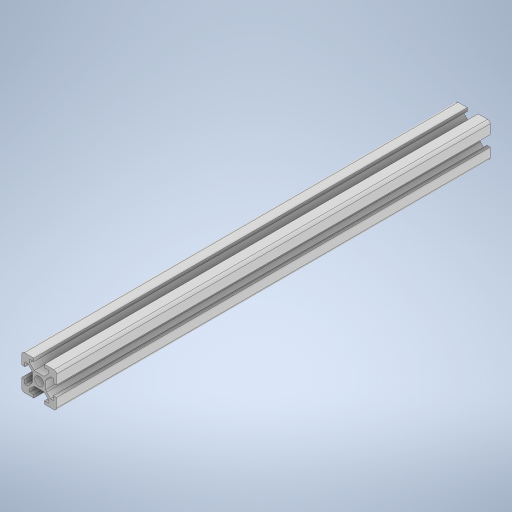
# Autodesk Inventor part: perfil_2020T
Saved by Autodesk Inventor 2023.2 (Build 272271030, 271C)
## iProperties
Created: 2023-03-04
Part Number: perfil_2020T
Material: Generic
Document SubType Name: Modeling
Designer: Cris Pat
Density: 1 g/cm^3
Appearance: Default
Author: Cris Pat
Autodesk Inventor part; units mm, degrees
ref_plane "YZ Plane" through (0, 0, 0) normal (1, 0, 0) x (0, 1, 0)
ref_plane "XZ Plane" through (0, 0, 0) normal (0, 1, 0) x (-1, 0, 0)
ref_plane "XY Plane" through (0, 0, 0) normal (0, 0, 1) x (1, 0, 0)
sketch "Sketch1" plane through (0, 0, 0) normal (0, 0, 1) x (1, 0, 0)
  line L0 (-10, 10) -> (10, 10) construction
  line L1 (10, 10) -> (10, -10) construction
  line L2 (10, -10) -> (-10, -10) construction
  line L3 (-10, -10) -> (-10, 10) construction
  line L4 (0, 10) -> (0, -10) construction
  circle A0 centre (0, 0) radius 2.5
  line L5 (10, 0) -> (-10, 0) construction
  line L6 (0, 0) -> (10, 10) construction
  line L7 (-3.9, 3.9) -> (3.9, 3.9) construction
  line L8 (3.9, 3.9) -> (3.9, -3.9) construction
  line L9 (3.9, -3.9) -> (-3.9, -3.9) construction
  line L10 (-3.9, -3.9) -> (-3.9, 3.9) construction
  line L11 (2.8393, 3.9) -> (3.9, 2.8393) construction
  line L12 (10, 10) -> (5.5, 10) construction
  line L13 (5.5, 10) -> (5.5, 5.5) construction
  line L14 (5.5, 5.5) -> (10, 5.5) construction
  line L15 (10, 5.5) -> (10, 10) construction
  line L16 (3.9, 0) -> (3.9, 2.8393)
  line L17 (3.9, 2.8393) -> (6.5607, 5.5)
  line L18 (0, 3.9) -> (2.8393, 3.9)
  line L19 (2.8393, 3.9) -> (5.5, 6.5607)
  line L20 (10, 10) -> (10, 3.1)
  line L21 (10, 3.1) -> (8.2, 3.1)
  line L22 (8.2, 3.1) -> (8.2, 5.5)
  line L23 (6.5607, 5.5) -> (8.2, 5.5)
  line L24 (10, 10) -> (3.1, 10)
  line L25 (3.1, 10) -> (3.1, 8.2)
  line L26 (3.1, 8.2) -> (5.5, 8.2)
  line L27 (5.5, 6.5607) -> (5.5, 8.2)
  line L28 (-3.9, 0) -> (-3.9, 2.8393)
  line L29 (-3.9, 2.8393) -> (-6.5607, 5.5)
  line L30 (0, 3.9) -> (-2.8393, 3.9)
  line L31 (-2.8393, 3.9) -> (-5.5, 6.5607)
  line L32 (-10, 10) -> (-10, 3.1)
  line L33 (-10, 3.1) -> (-8.2, 3.1)
  line L34 (-8.2, 3.1) -> (-8.2, 5.5)
  line L35 (-6.5607, 5.5) -> (-8.2, 5.5)
  line L36 (-10, 10) -> (-3.1, 10)
  line L37 (-3.1, 10) -> (-3.1, 8.2)
  line L38 (-3.1, 8.2) -> (-5.5, 8.2)
  line L39 (-5.5, 6.5607) -> (-5.5, 8.2)
  line L40 (3.9, 0) -> (3.9, -2.8393)
  line L41 (3.9, -2.8393) -> (6.5607, -5.5)
  line L42 (0, -3.9) -> (2.8393, -3.9)
  line L43 (2.8393, -3.9) -> (5.5, -6.5607)
  line L44 (10, -10) -> (10, -3.1)
  line L45 (10, -3.1) -> (8.2, -3.1)
  line L46 (8.2, -3.1) -> (8.2, -5.5)
  line L47 (6.5607, -5.5) -> (8.2, -5.5)
  line L48 (10, -10) -> (3.1, -10)
  line L49 (3.1, -10) -> (3.1, -8.2)
  line L50 (3.1, -8.2) -> (5.5, -8.2)
  line L51 (5.5, -6.5607) -> (5.5, -8.2)
  line L52 (-3.9, 0) -> (-3.9, -2.8393)
  line L53 (-3.9, -2.8393) -> (-6.5607, -5.5)
  line L54 (-6.5607, -5.5) -> (-8.2, -5.5)
  line L55 (-8.2, -3.1) -> (-8.2, -5.5)
  line L56 (-10, -3.1) -> (-8.2, -3.1)
  line L57 (-10, -10) -> (-10, -3.1)
  line L58 (-10, -10) -> (-3.1, -10)
  line L59 (-3.1, -10) -> (-3.1, -8.2)
  line L60 (-3.1, -8.2) -> (-5.5, -8.2)
  line L61 (-5.5, -6.5607) -> (-5.5, -8.2)
  line L62 (-2.8393, -3.9) -> (-5.5, -6.5607)
  line L63 (0, -3.9) -> (-2.8393, -3.9)
  point P0 (0, 0)
  point P1 (0, 0)
  dimension "d8" = 20
  dimension "d9" = 20
  dimension "d10" = 5
  dimension "d18" = 6.1
  dimension "d19" = 6.1
  dimension "d21" = 1.5
  dimension "d24" = 4.5
  dimension "d25" = 4.5
  dimension "d26" = 1.5
  dimension "d27" = 6.9
  dimension "d28" = 1.8
  constraints: 128 end point, 35 symmetric about line, 8 midpoint, 7 parallel, 6 perpendicular, 6 point on line, 3 horizontal, 2 collinear, 2 horizontal alignment, 2 vertical alignment, 1 centre point, 1 coincident, 1 vertical
  measures "d8" distance of L1.end L2.end
  measures "d9" distance of L0.end L1.end
  measures "d10" diameter of A0
  measures "d18" distance between parallel lines of L2 L9
  measures "d19" distance between parallel lines of L3 L10
  measures "d21" distance of L11.start L11.end
  measures "d24" distance between parallel lines of L1 L13
  measures "d25" distance between parallel lines of L0 L14
  measures "d26" distance between parallel lines of L17 L19
  measures "d27" distance of L0.end L20.end
  measures "d28" distance of L20.end L21.end
extrude "Extrusion1" add sketch "Sketch1" along normal mid plane 250
fillet "Fillet1" radius 1.5 8 edges at (10, 10, 0) (-10, 10, 0) (10, -10, 0) (-10, -10, 0) (3.9, 2.8393, 0) (3.9, -2.8393, 0) (-3.9, 2.8393, 0) (-3.9, -2.8393, 0)
body "Solid1"
